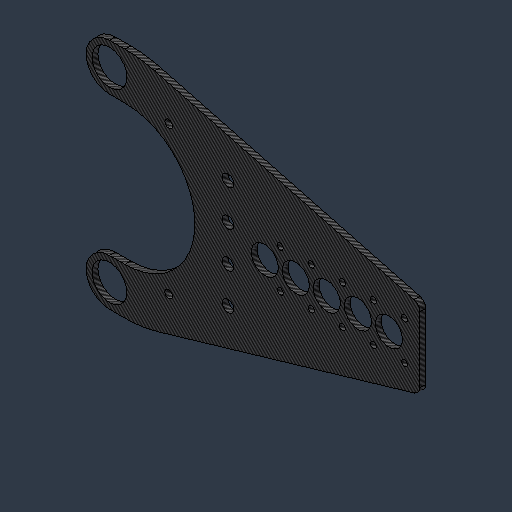
# Autodesk Inventor part: PLATE,END_EFFECTOR,ARM
Saved by Autodesk Inventor 2024.3 (Build 283343000, 343)
## iProperties
ILogicPurgeVersion: 0.0.0.0
OnSaveVersion: 3.5.0.0
OnSaveAssembly: COREAutomationManager
Category: _
Manager: _
Created: 2025-03-21
Part Number: PLATE,END_EFFECTOR,ARM
Checked By: 00
Engr Approved By: _
User Status: Work In Process
Material: Polycarbonate, Clear
Description: STANDARD (mm)
Document SubType Name: Sheet Metal
Mfg Approved By: John.Thibert
Designer: John Thibert
Manufacturer: Standard
Standards Organization: Custom
Density: 1.2 g/cm^3
Sheet Metal Rule: Default
Appearance: Carbon Fiber
Mass: 140.878 g
Surface Area: 576.784 cm^2
Volume: 117.398 cm^3
CN_MASS: 0.14
CN_SERVICEABLE: _
FIRST_DESCRIPTION: _
SECOND_DESCRIPTION: _
THIRD_DESCRIPTION: _
ModelCat: Uncategorized
MaterialName: Polycarbonate, Clear
Subject: _
Author: John Thibert
Keywords: -
Revision Number: A
Autodesk Inventor part; units mm, degrees
ref_plane "YZ Plane" through (0, 0, 0) normal (1, 0, 0) x (0, 1, 0)
ref_plane "XZ Plane" through (0, 0, 0) normal (0, 1, 0) x (-1, 0, 0)
ref_plane "XY Plane" through (0, 0, 0) normal (0, 0, 1) x (1, 0, 0)
sketch "Sketch2" plane through (0, 0, 0) normal (0, 0, 1) x (1, 0, 0)
  arc A0 (0, -57.15) -> (0, 57.15) centre (0, 0) ccw
  line L0 (241.3, 34.925) -> (241.3, -28.575)
  line L1 (-90.17, 0) -> (296.545, 0) construction
  arc A1 (0, -95.25) -> (26.7739, -91.4096) centre (0, 0) ccw
  arc A2 (24.2674, 92.1068) -> (0, 95.25) centre (0, 0) ccw
  line L2 (26.7739, -91.4096) -> (241.3, -28.575)
  line L3 (241.3, 34.925) -> (24.2674, 92.1068)
  line L4 (0, 95.25) -> (-12.7, 95.25)
  arc A3 (-12.7, 95.25) -> (-12.7, 57.15) centre (-12.7, 76.2) ccw
  line L5 (-12.7, 57.15) -> (0, 57.15)
  line L6 (0, -57.15) -> (-12.7, -57.15)
  arc A4 (-12.7, -57.15) -> (-12.7, -95.25) centre (-12.7, -76.2) ccw
  line L7 (-12.7, -95.25) -> (0, -95.25)
  circle A5 centre (-12.7, -76.2) radius 22.225 construction
  circle A6 centre (-12.7, 76.2) radius 22.225 construction
  line L8 (0, 137.795) -> (0, -137.795) construction
  point P0 (57.15, 0)
  point P1 (241.3, 3.175)
  dimension "d0" = 114.3
  dimension "d1" = 63.5
  dimension "d20" = 12.7
  dimension "d21" = 19.05
  dimension "d63" = 44.45
  dimension "d65" = 57.15
  dimension "d73" = 241.3
  dimension "d78" = 3.175
  measures "d0" diameter of A0
  measures "d1" distance of L0.start L0.end
  measures "d20" distance of L4.start L4.end
  measures "d21" radius of A3
  measures "d63" diameter of A5
  measures "d65" distance from line of point (57.15, 0) L8
  measures "d73" distance from line of L0 A0.centre
  measures "d78" distance from line of L1 point (241.3, 3.175)
extrude "Plate1" add sketch "Sketch2" along normal blind 4.7625
sketch "Sketch3" plane through (0, 0, 4.7625) normal (0, 0, 1) x (1, 0, 0)
  line L0 (241.3, 34.925) -> (241.3, -28.575) construction
  line L1 (-86.36, 0) -> (295.91, 0) construction
  line L2 (228.6, 19.05) -> (228.6, -12.7) construction
  point P0 (0, 0)
  dimension "d7" = 31.75
  dimension "d8" = 12.7
  dimension "d75" = 19.05
  constraints: 2 coincident, 2 end point, 1 vertical
  measures "d7" distance of L2.start L2.end
  measures "d8" distance between parallel lines of L0 L2
  measures "d75" distance from line of L1 L2.start
hole "Hole1" at (228.6, 19.05, 4.7625) at (228.6, -12.7, 4.7625) direction (0, 0, -1) diameter 5.1054 end through all clearance for "Flat Head Machine Screw (82)" size "#10" standard "Ansi Unified Screw Threads"
pattern_linear "Rectangular Pattern1" count 5 spacing 25.4 along (-1, 0, 0) of "Hole1"
sketch "Sketch4" plane through (0, 0, 4.7625) normal (0, 0, 1) x (1, 0, 0)
  arc A0 (-12.7, 95.25) -> (-12.7, 57.15) centre (-12.7, 76.2) ccw construction
  arc A1 (-12.7, -57.15) -> (-12.7, -95.25) centre (-12.7, -76.2) ccw construction
  line L0 (-12.7, 76.2) -> (84.2314, 44.45) construction
  line L1 (-86.36, 0) -> (295.91, 0) construction
  line L2 (-12.7, -76.2) -> (84.2314, -44.45) construction
  circle A2 centre (84.2314, 44.45) radius 11.43 construction
  circle A3 centre (-12.7, 76.2) radius 11.43 construction
  line L3 (-9.1421, 87.0621) -> (87.7893, 55.3121) construction
  line L4 (-16.2579, 65.3379) -> (80.6735, 33.5879) construction
  line L5 (84.2314, 14.8167) -> (84.2314, -14.8167) construction
  point P0 (0, 0)
  point P1 (-12.7, -76.2)
  point P2 (84.2314, 0)
  dimension "d29" = 101.9988
  dimension "d30" = 44.45
  dimension "d38" = 22.86
  dimension "d39" = 29.6333
  dimension "d40" = 29.6333
  dimension "d41" = 29.6333
  constraints: 10 end point, 8 coincident, 4 point on circle, 3 symmetric about line, 3 tangent, 2 centre point, 2 point on line, 1 equal radius, 1 midpoint, 1 parallel, 1 vertical
  measures "d29" distance of L0.start L0.end
  measures "d30" distance from line of L1 L0.end
  measures "d38" diameter of A2
  measures "d39" distance of point (84.231, 44.45) L5.start
  measures "d40" distance of L5.start L5.end
  measures "d41" distance of L2.end point (84.231, -14.817)
hole "Hole2" at (-12.7, 76.2, 4.7625) at (-12.7, -76.2, 4.7625) direction (0, 0, -1) diameter 28.575 end through all
hole "Hole3" at (84.2314, 44.45, 4.7625) at (84.2314, -44.45, 4.7625) at (84.2314, 14.8167, 4.7625) at (84.2314, -14.8167, 4.7625) direction (0, 0, -1) diameter 9.525 end through all
sketch "Sketch5" plane through (0, 0, 4.7625) normal (0, 0, 1) x (1, 0, 0)
  arc A0 (0, -57.15) -> (0, 57.15) centre (0, 0) ccw construction
  line L0 (-12.7, -57.15) -> (0, -57.15) construction
  arc A1 (-12.7, -57.15) -> (-12.7, -95.25) centre (-12.7, -76.2) ccw construction
  line L1 (0, -95.25) -> (-12.7, -95.25) construction
  arc A2 (0, -95.25) -> (26.7739, -91.4096) centre (0, 0) ccw construction
  line L2 (241.3, -28.575) -> (26.7739, -91.4096) construction
  line L3 (0, 57.15) -> (-12.7, 57.15) construction
  arc A3 (-12.7, 95.25) -> (-12.7, 57.15) centre (-12.7, 76.2) ccw construction
  line L4 (-12.7, 95.25) -> (0, 95.25) construction
  arc A4 (24.2674, 92.1068) -> (0, 95.25) centre (0, 0) ccw construction
  line L5 (24.2674, 92.1068) -> (241.3, 34.925) construction
  line L6 (197.4777, 33.3375) -> (105.4027, 57.5966)
  arc A5 (21.0318, 79.8259) -> (12.7, 81.5672) centre (0, 0) ccw
  arc A6 (69.85, 0) -> (53.5082, 44.8987) centre (0, 0) ccw construction
  line L7 (77.4255, 64.9677) -> (53.5082, 44.8987)
  line L8 (12.7, 81.5672) -> (12.7, 68.6858)
  line L9 (-86.36, 0) -> (295.91, 0) construction
  line L10 (241.3, 34.925) -> (241.3, -28.575) construction
  arc A7 (53.5082, 44.8987) -> (12.7, 68.6858) centre (0, 0) ccw
  line L11 (77.4255, 64.9677) -> (21.0318, 79.8259)
  line L12 (105.4027, 57.5966) -> (105.4027, 33.3375)
  line L13 (105.4027, 33.3375) -> (197.4777, 33.3375)
  line L14 (105.4027, 57.5966) -> (77.4255, 64.9677) construction
  line L15 (105.4027, -55.1457) -> (201.5387, -26.9875)
  line L16 (201.5387, -26.9875) -> (105.4027, -26.9875)
  line L17 (105.4027, -26.9875) -> (105.4027, -55.1457)
  circle A8 centre (152.4, 19.05) radius 2.5527 construction
  circle A9 centre (152.4, -12.7) radius 2.5527 construction
  point P0 (0, 0)
  dimension "d42" = 12.7
  dimension "d43" = 12.7
  dimension "d44" = 25.4
  dimension "d45" = 50
  dimension "d47" = 33.3375
  dimension "d48" = 92.075
  dimension "d66" = 12.7
  dimension "d67" = 26.9875
  dimension "d76" = 14.2875
  dimension "d77" = 14.2875
  constraints: 20 end point, 6 point on circle, 3 centre point, 3 collinear, 2 perpendicular, 2 point on line, 1 horizontal, 1 parallel, 1 tangent, 1 vertical
  measures "d42" distance between parallel lines of L5 L6
  measures "d43" radial gap between concentric circles of A0 A6
  measures "d44" distance from line of L8 A3.centre
  measures "d45" angle of L7 L8
  measures "d47" distance between parallel lines of L9 L13
  measures "d48" distance of L6.start L12.end
  measures "d66" distance between parallel lines of L2 L15
  measures "d67" distance between parallel lines of L9 L16
  measures "d76" distance from line of L13 A8.centre
  measures "d77" distance from line of L16 A9.centre
cut "Cut1" [suppressed]
cut "Cut2" [suppressed]
sketch "Sketch6" plane through (0, 0, 4.7625) normal (0, 0, 1) x (1, 0, 0)
  circle A0 centre (228.6, 19.05) radius 2.5527 construction
  circle A1 centre (203.2, -12.7) radius 2.5527 construction
  line L0 (228.6, 19.05) -> (203.2, -12.7) construction
  point P0 (0, 0)
  point P1 (215.9, 3.175)
  constraints: 2 end point, 1 midpoint
hole "Hole4" at (215.9, 3.175, 4.7625) direction (0, 0, -1) diameter 22.225 end through all
pattern_linear "Rectangular Pattern2" count 5 spacing 25.4 along (-1, 0, 0) of "Hole4"
feature "Corner Round1" [suppressed]
mirror "Mirror2" [suppressed]
sketch "Sketch7" plane through (0, 0, 4.7625) normal (0, 0, 1) x (1, 0, 0)
  circle A0 centre (-12.7, 76.2) radius 14.2875 construction
  circle A1 centre (-12.7, -76.2) radius 14.2875 construction
  circle A2 centre (84.2314, -44.45) radius 4.7625 construction
  circle A3 centre (84.2314, 44.45) radius 4.7625 construction
  line L0 (84.2314, 44.45) -> (-12.7, 76.2) construction
  line L1 (-12.7, -76.2) -> (84.2314, -44.45) construction
  line L2 (59.9985, 52.3875) -> (64.9401, 67.4738) construction
  line L3 (59.9985, -52.3875) -> (64.9401, -67.4738) construction
  point P0 (0, 0)
  point P1 (35.7657, 60.325)
  point P2 (35.7657, -60.325)
  dimension "d86" = 25.4997
  dimension "d87" = 50.9994
  dimension "d88" = 25.4997
  dimension "d89" = 15.875
  constraints: 8 end point, 2 coincident, 2 midpoint, 2 perpendicular, 2 point on line, 1 equal length
  measures "d86" distance from line of point (35.766, 60.325) L2
  measures "d87" distance of L0.start point (35.766, 60.325)
  measures "d88" distance from line of point (35.766, -60.325) L3
  measures "d89" distance of L2.start L2.end
hole "Hole5" at (35.7657, 60.325, 4.7625) at (35.7657, -60.325, 4.7625) direction (0, 0, -1) diameter 6.35 end through all
fillet "Corner Round3" radius 6.35 2 edges at (241.3, -28.575, 2.3813) (241.3, 34.925, 2.3813)
equation "\"d14\" = Thickness"
equation "\"d39\" = d40"
equation "\"d66\" = d42"
equation "\"d86\" = 0.5 * d87"
equation "\"d88\" = d86"
equation "\"d49\" = Thickness"
equation "\"d68\" = Thickness"
equation "\"d84\" = Thickness"
equation "\"d6\" = Thickness"
equation "\"BendRadius\" = 1.5 * Thickness"
equation "\"BendReliefWidth\" = Thickness"
equation "\"BendReliefDepth\" = 0.5 * Thickness"
equation "\"CornerReliefSize\" = 4 * Thickness"
equation "\"MinimumRemnant\" = 2 * Thickness"
equation "\"TransitionRadius\" = BendRadius"
equation "\"JacobiRadiusSize\" = BendRadius"
equation "\"GapSize\" = Thickness"
equation "\"Thickness\" = 4.7625"
body "Solid1"
